VIHALS Controller Top Wire Holder (Autodesk Fusion 360 design; units mm, degrees)
Autodesk Fusion 360 part; units mm, degrees
note: some values were not read from the file. Set by a fixed rule: which sketch regions a step uses.
sketch "Sketch1" plane through (0, 0, 0) normal (0, 0, 1) x (1, 0, 0)
  line L0 (-12.5, 10) -> (12.5, 10)
  line L1 (12.5, 10) -> (12.5, -10)
  line L2 (12.5, -10) -> (-12.5, -10)
  line L3 (-12.5, -10) -> (-12.5, 10)
  dimension "d1" = 20
  dimension "d2" = 25
  dimension "d3" = 12.5
  dimension "d4" = 10
  constraint horizontal L0
  constraint vertical L1
  constraint horizontal L2
  constraint vertical L3
  measures "d1" distance of L0 L2
  measures "d2" distance of L1 L3
  measures "d3" distance of origin L3
  measures "d4" distance of origin L2
extrude "Extrude1" add sketch "Sketch1" along normal blind 3
sketch "Sketch3" plane through (0, 0, 3) normal (0, 0, 1) x (-1, 0, 0)
  line L0 (12.5, -10) -> (12.5, 10)
  line L1 (12.5, 10) -> (-12.5, 10)
  line L2 (-12.5, 10) -> (-12.5, -10)
  line L3 (-12.5, -10) -> (12.5, -10)
  point P0 (3, -4)
  point P1 (-7, 4)
  dimension "d32" = 5.5
  dimension "d33" = 4
  dimension "d34" = 4
  dimension "d41" = 10
  measures "d32" distance of L2 P1
  measures "d33" vertical distance of origin P1
  measures "d34" vertical distance of origin P0
  measures "d41" horizontal distance of P0 P1
hole "Hole2" at (-3, 4, 3) at (7, -4, 3) direction (0, 0, -1) diameter 3.797 depth 6 tip angle 118 countersink diameter 7.087 countersink angle 100
sketch "Sketch4" plane through (0, 0, 3) normal (0, 0, 1) x (-1, 0, 0)
  circle A0 centre (3, -4) radius 3.5435
  circle A1 centre (-7, 4) radius 3.5435
  line L0 (12.5, 10) -> (-12.5, 10)
  line L1 (-12.5, 10) -> (-12.5, -10)
  line L2 (-12.5, -10) -> (12.5, -10)
  line L3 (12.5, -10) -> (12.5, 10)
  circle A2 centre (18, 0.375) radius 1.5
  circle A3 centre (18, -0.375) radius 1.5
  circle A4 centre (18, 0.375) radius 2.75
  circle A5 centre (18, -0.375) radius 2.75
  line L4 (18, 0.375) -> (17.0157, 0.375)
  line L5 (17.0157, 0.375) -> (17.0157, -0.375)
  line L6 (17.0157, -0.375) -> (18, -0.375)
  line L7 (18, -0.375) -> (18, 0.375)
  line L8 (18, -0.375) -> (24.9519, -0.375)
  line L9 (24.9519, -0.375) -> (24.9519, 0.375)
  line L10 (24.9519, 0.375) -> (18, 0.375)
  line L11 (18, 0.375) -> (18, -0.375)
  line L12 (16.5, 5) -> (16.5, -5)
  line L13 (16.5, 5) -> (12.5, 10)
  line L14 (16.5, -5) -> (12.5, -10)
  dimension "d44" = 3
  dimension "d45" = 3
  dimension "d46" = 5.5
  dimension "d47" = 5.5
  dimension "d48" = 0.75
  dimension "d49" = 0.375
  dimension "d50" = 1.5
  dimension "d51" = 10
  dimension "d52" = 5
  dimension "d55" = 4
  constraint vertical A2.centre A3.centre
  constraint concentric A2 A4
  constraint concentric A3 A5
  constraint horizontal L4
  constraint vertical L5
  constraint horizontal L6
  constraint vertical L7
  constraint coincident A2.centre A4.centre
  constraint horizontal L8
  constraint vertical L9
  constraint horizontal L10
  constraint vertical L11
  constraint coincident A3.centre A5.centre
  constraint horizontal L4.end L9.end
  constraint horizontal L5.end L8.end
  constraint vertical L12
  constraint coincident L0.start L3.end
  constraint coincident L2.end L3.start
  measures "d44" diameter of A2
  measures "d45" diameter of A3
  measures "d46" diameter of A4
  measures "d47" diameter of A5
  measures "d48" distance of A2.centre A3.centre
  measures "d49" vertical distance of origin A2.centre
  measures "d50" distance of A2.centre L12
  measures "d51" distance of L12.start L12.end
  measures "d52" vertical distance of origin L12.end
  measures "d55" distance of L3 L12
extrude "Extrude4" add sketch "Sketch4" against normal blind 3 contours L3 A4 A5 L12 L13 L14 | A4 A5 L12 | A4 A5 L10 L12 | A4 A5 L8 L12 | A4 A5 L12 | A4 A5 L12 | A2 A5 L10 L12 | A3 A4 L8 L12
fillet "Fillet3" radius 15 2 edges at (-16.5, -2.6799, 1.5) (-16.5, 2.6799, 1.5)
fillet "Fillet3" radius 0.25 2 edges at (-20.75, 0.375, 1.5) (-20.75, -0.375, 1.5)
fillet "Fillet3" radius 2 2 edges at (-16.5, 5, 1.5) (-16.5, -5, 1.5)
equation "d49 = ( 0.75 / 2 ) * 1 mm"
